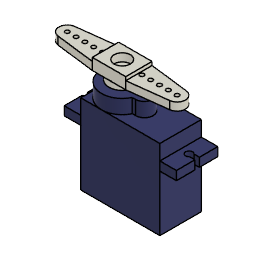
Servo Motor SG90 (Autodesk Fusion 360 design; units mm, degrees)
Autodesk Fusion 360 part; units mm, degrees
sketch "Sketch1" plane through (0, 0, 0) normal (0, 0, 1) x (1, 0, 0)
  circle A0 centre (0, 0) radius 2.3
  circle A1 centre (0, 0) radius 5.9
  line L0 (5.9, 5.9) -> (-5.9, 5.9) construction
  line L1 (-5.9, 5.9) -> (-5.9, -5.9) construction
  line L2 (-5.9, -5.9) -> (5.9, -5.9) construction
  line L3 (5.9, -5.9) -> (5.9, 5.9) construction
  line L4 (5.9, 5.9) -> (-5.9, -5.9) construction
  line L5 (-5.9, 5.9) -> (5.9, -5.9) construction
  line L6 (-5.9, 5.9) -> (16.6, 5.9)
  line L7 (16.6, 5.9) -> (16.6, -5.9)
  line L8 (16.6, -5.9) -> (-5.9, -5.9)
  line L9 (-5.9, -5.9) -> (-5.9, 5.9)
  circle A2 centre (6.3, 0) radius 2.5
  line L10 (6.3, 2.5) -> (5.3442, 2.5)
  line L11 (6.3, -2.5) -> (5.3442, -2.5)
  line L12 (5.35, 7) -> (5.35, -7) construction
  line L13 (-5.9, 5.9) -> (-10.6, 5.9)
  line L14 (-10.6, 5.9) -> (-10.6, 0.65)
  line L15 (-10.6, 0.65) -> (-8.3, 0.65)
  line L16 (-8.3, 0.65) -> (-8.3, -0.65)
  line L17 (-8.3, -0.65) -> (-10.6, -0.65)
  line L18 (-10.6, -0.65) -> (-10.6, -5.9)
  line L19 (-10.6, -5.9) -> (-5.9, -5.9)
  circle A3 centre (-8.3, 0) radius 1
  line L20 (16.6, 5.9) -> (21.3, 5.9)
  line L21 (21.3, 5.9) -> (21.3, 0.65)
  line L22 (21.3, 0.65) -> (19, 0.65)
  circle A4 centre (19, 0) radius 1
  line L23 (19, -0.65) -> (21.3, -0.65)
  line L24 (21.3, -0.65) -> (21.3, -5.9)
  line L25 (21.3, -5.9) -> (16.6, -5.9)
  dimension "d1" = 4.6
  dimension "d2" = 11.8
  dimension "d3" = 11.8
  dimension "d4" = 11.8
  dimension "d5" = 22.5
  dimension "d6" = 11.8
  dimension "d7" = 5
  dimension "d8" = 10.3
  dimension "d9" = 11.25
  dimension "d10" = 4.7
  dimension "d11" = 5.25
  dimension "d12" = 2.3
  dimension "d13" = 1.3
  dimension "d14" = 2
  constraint coincident A0.centre A1.centre
  constraint concentric A0 A1
  constraint horizontal L0
  constraint perpendicular L0 L1
  constraint parallel L0 L2
  constraint parallel L1 L3
  constraint coincident L4 A0.centre
  constraint coincident L5 A0.centre
  constraint horizontal L6
  constraint vertical L7
  constraint horizontal L8
  constraint vertical L9
  constraint coincident A2 L10.start
  constraint coincident A1 L10.end
  constraint perpendicular L3 L10
  constraint coincident A2 L11.start
  constraint coincident A1 L11.end
  constraint tangent A2 L11
  constraint perpendicular L3 L11
  constraint perpendicular L8 L12
  constraint perpendicular L9 L13
  constraint perpendicular L13 L14
  constraint perpendicular L14 L15
  constraint perpendicular L15 L16
  constraint perpendicular L16 L17
  constraint perpendicular L2 L18
  constraint perpendicular L9 L19
  constraint midpoint L16 A3.centre
  constraint symmetric L0.end L12 L6.end
  constraint symmetric L1.end L12 L7.end
  constraint symmetric L12 L13.end L20.end
  constraint symmetric L12 L14.end L21.end
  constraint symmetric L12 L15.end L22.end
  constraint symmetric L12 L16.end L23.start
  constraint symmetric L12 L17.end L23.end
  constraint symmetric L12 L18.end L24.end
  constraint symmetric L12 A3 A4
  measures "d1" diameter of A0
  measures "d2" diameter of A1
  measures "d3" distance of L1.end L2.end
  measures "d4" distance of L0.end L1.end
  measures "d5" distance of L0.end L6.end
  measures "d6" distance of L0.end L1.end
  measures "d7" diameter of A2
  measures "d8" distance of L7 A2.centre
  measures "d9" distance of L7 L12
  measures "d10" distance of L0.end L13.end
  measures "d11" distance of L13.end L14.end
  measures "d12" distance of L14.end L15.end
  measures "d13" distance of L15.end L16.end
  measures "d14" diameter of A3
extrude "Extrude1" add sketch "Sketch1" along normal blind 22.7 contours A0 | A1 A2 | A1 A2 | A1 A2 | A1 A2 L10 | A1 A2 L11 | A1 L6 L7 L8 A2 L10 L11 | A1 L6 L9 | A1 L8 L9 makes body 1 in component "Housing"
extrude "Extrude2" add sketch "Sketch1" along normal blind 4 from surface at 22.7 contours A1 A2 | A1 A2 | A1 A2 | A1 A2 L10 | A1 A2 L11 bodies 1 in component "Housing"
extrude "Extrude3" add sketch "Sketch1" along normal blind 2.5 from surface at 15.9 separate body contours L9 L13 L14 L15 L17 L18 L19 A3 | L7 L20 L21 L22 A4 L23 L24 L25 makes body 2 at (18.9594, -4.2666, 15.9) makes body 3 at (-8.2594, -4.2666, 15.9) in component "Housing"
extrude "Extrude1'" add sketch "Sketch1" along normal blind 7.2 from surface at 22.7 separate body contours A0 makes body 4 in component "Shaft"
sketch "Sketch2" plane through (-5.9, 0, 0) normal (-1, 0, 0) x (0, -1, 0)
  line L0 (-5.9, 22.7) -> (-5.9, 0)
  line L1 (-5.9, 0) -> (5.9, 0)
  line L2 (5.9, 0) -> (5.9, 22.7)
  line L3 (0, 0) -> (-1.75, 0) construction
  line L4 (-1.75, 0) -> (1.75, 0)
  line L5 (1.75, 0) -> (1.75, 4.5)
  line L6 (1.75, 4.5) -> (-1.75, 4.5)
  line L7 (-1.75, 4.5) -> (-1.75, 0)
  line L8 (5.9, 22.7) -> (0, 22.7)
  line L9 (0, 22.7) -> (-5.9, 22.7)
  dimension "d26" = 1.75
  dimension "d27" = 3.5
  dimension "d28" = 4.5
  constraint coincident L3.start origin
  constraint parallel L1 L3
  constraint horizontal L4
  constraint vertical L5
  constraint horizontal L6
  constraint vertical L7
  measures "d26" distance of L3.start L3.end
  measures "d27" distance of L3.end L4.end
  measures "d28" distance of L3.end L6.end
extrude "Extrude4" cut sketch "Sketch2" against normal blind 1.5 contours L1 L4 L5 L6 L7 bodies 1 2 3 in component "Housing"
sketch "Sketch1 (2)" plane through (0, 0, 22.7) normal (0, 0, -1) x (1, 0, 0) in component "Arm"
  circle A0 centre (0, 0) radius 2.3
  circle A1 centre (0, 0) radius 3.75
  arc A2 (-1.95, -7.5) -> (1.95, -7.5) centre (0, -7.5) ccw
  arc A3 (1.95, 7.5) -> (-1.95, 7.5) centre (0, 7.5) ccw
  line L0 (0, 7.5) -> (0, -7.5) construction
  line L1 (4.75, 3.75) -> (-4.75, 3.75)
  line L2 (-4.75, 3.75) -> (-4.75, -3.75)
  line L3 (-4.75, -3.75) -> (4.75, -3.75)
  line L4 (4.75, -3.75) -> (4.75, 3.75)
  line L5 (4.75, 3.75) -> (-4.75, -3.75) construction
  line L6 (-4.75, 3.75) -> (4.75, -3.75) construction
  arc A4 (15.8924, -2.3821) -> (15.8924, 2.3821) centre (15.6, 0) ccw
  arc A5 (-15.8924, 2.3821) -> (-15.8924, -2.3821) centre (-15.6, 0) ccw
  line L7 (-18, 0) -> (18, 0) construction
  line L8 (-4.75, 3.75) -> (-15.8924, 2.3821)
  line L9 (-4.75, -3.75) -> (-15.8924, -2.3821)
  line L10 (4.75, -3.75) -> (15.8924, -2.3821)
  line L11 (4.75, 3.75) -> (15.8924, 2.3821)
  circle A6 centre (0, 7.5) radius 0.6
  circle A7 centre (0, 5) radius 0.6
  circle A8 centre (0, -5) radius 0.6
  circle A9 centre (0, -7.5) radius 0.6
  circle A10 centre (-15.6, 0) radius 0.6
  circle A11 centre (-13.1, 0) radius 0.6
  circle A12 centre (-10.6, 0) radius 0.6
  circle A13 centre (-8.1, 0) radius 0.6
  circle A14 centre (-5.6, 0) radius 0.6
  circle A15 centre (5.6, 0) radius 0.6
  circle A16 centre (8.1, 0) radius 0.6
  circle A17 centre (10.6, 0) radius 0.6
  circle A18 centre (13.1, 0) radius 0.6
  circle A19 centre (15.6, 0) radius 0.6
  line L12 (-1.95, 7.5) -> (-1.95, 3.75)
  line L13 (-1.95, -3.75) -> (-1.95, -7.5)
  line L14 (1.95, -7.5) -> (1.95, -3.75)
  line L15 (1.95, 3.75) -> (1.95, 7.5)
  dimension "d37" = 7.5
  dimension "d38" = 3.9
  dimension "d39" = 9.5
  dimension "d40" = 7.5
  dimension "d41" = 36
  dimension "d42" = 4.8
  dimension "d43" = 1.2
  dimension "d46" = 0
  dimension "d47" = -2.5
  dimension "d48" = 1.2
  dimension "d51" = 10
  dimension "d52" = 0
  constraint coincident A0.centre A1.centre
  constraint tangent A2 L13
  constraint tangent A2 L14
  constraint parallel L12 L15
  constraint tangent A3 L15
  constraint tangent A3 L12
  constraint vertical L0
  constraint horizontal L1
  constraint perpendicular L1 L2
  constraint parallel L1 L3
  constraint parallel L2 L4
  constraint coincident L5 A0.centre
  constraint coincident L6 A0.centre
  constraint perpendicular L7 L13
  constraint tangent A5 L8
  constraint tangent A5 L9
  constraint tangent A4 L10
  constraint tangent A4 L11
  constraint coincident A5 L7.start
  constraint coincident A4 L7.end
  constraint concentric A3 A6
  constraint symmetric L7 A6 A9
  constraint symmetric L7 A7 A8
  constraint concentric A5 A10
  constraint symmetric L0 A10 A19
  constraint symmetric L0 A11 A18
  constraint symmetric L0 A12 A17
  constraint symmetric L0 A13 A16
  constraint symmetric L0 A14 A15
  constraint coincident L1 L12.end
  constraint collinear L12 L13
  constraint coincident L3 L13.start
  constraint coincident L3 L14.end
  constraint collinear L14 L15
  constraint coincident L1 L15.start
  measures "d37" diameter of A1
  measures "d38" diameter of A2
  measures "d39" distance of L2.end L3.end
  measures "d40" distance of L1.end L2.end
  measures "d41" distance of L7.start L7.end
  measures "d42" diameter of A4
  measures "d43" diameter of A6
  measures "d48" diameter of A10
extrude "Extrude1''" add sketch "Sketch1 (2)" along normal blind 2.25 and the other way blind 2.75 separate body contours A1 makes body 5 in component "Arm"
extrude "Extrude2'" add sketch "Sketch1 (2)" along normal up to surface (2.25 mm away) contours A1 L1 L3 L4 | A1 L1 L2 L3 bodies 5 in component "Arm"
extrude "Extrude3'" add sketch "Sketch1 (2)" along normal blind 1.25 and the other way blind 1 contours A1 L1 L3 L4 | A1 L1 L2 L3 | L4 A4 L10 L11 | L2 A5 L8 L9 bodies 5 in component "Arm"
component "Housing" placed x (1, 0, 0) y (0, 1, 0) z (0, 0, 1) at (0, 0, 0)
component "Shaft" placed x (1, 0, 0) y (0, -1, 0) z (0, 0, -1) at (0, 0, 52.6)
component "Arm" placed x (1, 0, 0) y (0, 1, 0) z (0, 0, 1) at (0, 0, 0) in component "Shaft"
equation "d26 = ( 3.5 / 2 ) * 1 mm"
equation "d51 = ( 2.5 * 4 ) * 1 mm"
